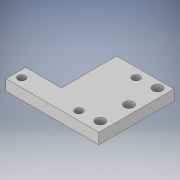
# Autodesk Inventor part: КВ33.044.407 - Заглушка разъема
Saved by Autodesk Inventor 2019 (Build 230136000, 136)
## iProperties
Created: 2019-11-19
Part Number: КВ33.044.407 - Заглушка разъема
Material: Типовые
Document SubType Name: Modeling
Designer: Петров Иван
Density: 1 g/cm^3
Appearance: По умолчанию
Author: Петров Иван
Autodesk Inventor part; units mm, degrees
ref_plane "YZ Plane" through (0, 0, 0) normal (1, 0, 0) x (0, 1, 0)
ref_plane "XZ Plane" through (0, 0, 0) normal (0, 1, 0) x (-1, 0, 0)
ref_plane "XY Plane" through (0, 0, 0) normal (0, 0, 1) x (1, 0, 0)
sketch "Эскиз1" plane through (0, 0, 0) normal (0, 1, 0) x (-1, 0, 0)
  circle A0 centre (-10.2546, 8.7513) radius 1.3
  circle A1 centre (-4.7546, 9.2513) radius 1.05
  circle A2 centre (-10.2546, 0.7513) radius 1.3
  circle A3 centre (-10.2546, -7.2487) radius 1.3
  circle A4 centre (-4.7546, -6.7487) radius 1.05
  circle A5 centre (11.2454, 9.2513) radius 1.05
  line L0 (-6.7546, 3.1513) -> (13.2454, 3.1513)
  line L1 (-6.7546, -3.3987) -> (-6.7546, 3.1513)
  line L2 (13.2454, -3.3987) -> (-6.7546, -3.3987)
  line L3 (13.2454, 3.1513) -> (13.2454, -3.3987)
  line L4 (3.2454, 3.1513) -> (3.2454, 6.1513)
  line L5 (3.2454, 6.1513) -> (13.2454, 6.1513)
  line L6 (13.2454, 6.1513) -> (13.2454, 11.6513)
  line L7 (13.2454, 11.6513) -> (-12.7546, 11.6513)
  line L8 (-12.7546, 11.6513) -> (-12.7546, -9.3487)
  line L9 (-12.7546, -9.3487) -> (3.2454, -9.3487)
  line L10 (3.2454, -3.3987) -> (3.2454, -6.3987)
  line L11 (3.2454, -6.3987) -> (3.2454, -9.3487)
  line L12 (3.2454, 3.1513) -> (3.2454, -3.3987)
  point P0 (0, 0)
  dimension "d0" = 3
  dimension "d1" = 5.5
  dimension "d2" = 26
  dimension "d3" = 21
  dimension "d4" = 3
  constraints: 26 end point, 6 centre point, 5 perpendicular, 3 vertical, 2 midpoint, 1 horizontal
  measures "d0" distance of L4.start L4.end
  measures "d1" distance of L5.end L6.end
  measures "d2" distance of L6.end L7.end
  measures "d3" distance of L7.end L8.end
  measures "d4" distance of L10.start L10.end
extrude "Выдавливание1" add sketch "Эскиз1" along normal blind 3 contours L1 L2 L10 L11 L9 L8 L7 L6 L5 L4 L0 | L0 L12 L2 L1
